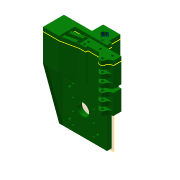
# Autodesk Inventor part: cellSTORM_cellphone_objectivelens_mount_flexure
Saved by Autodesk Inventor 2019 (Build 230136000, 136)
## iProperties
Created: 2020-02-11
Part Number: cellSTORM_cellphone_objectivelens_mount_flexure
Material: Generic
Document SubType Name: Modeling
Designer: diederichbenedict
Density: 1 g/cm^3
Appearance: Dark Green
Author: diederichbenedict
Autodesk Inventor part; units mm, degrees
ref_plane "YZ Plane" through (0, 0, 0) normal (1, 0, 0) x (0, 1, 0)
ref_plane "XZ Plane" through (0, 0, 0) normal (0, 1, 0) x (-1, 0, 0)
ref_plane "XY Plane" through (0, 0, 0) normal (0, 0, 1) x (1, 0, 0)
ref_plane "Work Plane1" through (0, 0, 0) normal (0, 0, 1) x (1, 0, 0)
sketch "Sketch1" plane through (0, 0, 0) normal (0, 0, 1) x (1, 0, 0)
  line L0 (28, 30) -> (30, 28) projected
  line L1 (28, 30) -> (-28, 30) projected
  line L2 (-30, 28) -> (-28, 30) projected
  line L3 (-30, 28) -> (-30, -28) projected
  line L4 (-28, -30) -> (-30, -28) projected
  line L5 (-28, -30) -> (28, -30) projected
  line L6 (30, -28) -> (28, -30) projected
  line L7 (30, -28) -> (30, 28) projected
  circle A0 centre (-17.5, -17.5) radius 1.95 projected
  circle A1 centre (17.5, 17.5) radius 1.95 projected
  circle A2 centre (17.5, -17.5) radius 1.95 projected
  circle A3 centre (-17.5, 17.5) radius 1.95 projected
  circle A4 centre (0, 0) radius 7.5 projected
  line L8 (-30, -30) -> (30, -30)
  line L9 (30, -30) -> (30, 30)
  line L10 (30, 30) -> (-30, 30)
  line L11 (-30, 30) -> (-30, -30)
  line L12 (30, 30) -> (-30, 30)
  line L13 (-30, 30) -> (-30, 45)
  line L14 (-30, 45) -> (30, 45)
  line L15 (30, 45) -> (30, 30)
  circle A5 centre (-13, 22.5) radius 1.45
  circle A6 centre (-13, 7.5) radius 1.45
  circle A7 centre (-13, -7.5) radius 1.45
  circle A8 centre (-13, -22.5) radius 1.45
  circle A9 centre (13, -22.5) radius 1.45
  circle A10 centre (13, 22.5) radius 1.45
  circle A11 centre (13, 7.5) radius 1.45
  circle A12 centre (13, -7.5) radius 1.45
  point P0 (0, 0)
  dimension "d2" = 60
  dimension "d3" = 15
  constraints: 16 end point, 8 centre point, 4 parallel, 2 horizontal, 2 perpendicular, 16 other
  measures "d2" distance of L13.end L14.end
  measures "d3" distance of L12.end L13.end
extrude "Extrusion1" add sketch "Sketch1" along normal blind 6
sketch "Sketch2" plane through (-30, 45, 0) normal (0, 1, 0) x (1, 0, 0)
  line L0 (60, 0) -> (0, 0) projected
  line L1 (0, 0) -> (0, -6) projected
  line L2 (60, -6) -> (0, -6) projected
  line L3 (60, 0) -> (60, -6) projected
  line L4 (0, 0) -> (0, -6) projected
  line L5 (0, 0) -> (19.8609, 0)
  line L6 (19.8609, 0) -> (19.8609, -26.2545)
  line L7 (19.8609, 0) -> (60, 0)
  line L8 (60, 0) -> (60, -6)
  line L9 (60, -6) -> (19.8609, -6)
  line L10 (19.8609, -6) -> (19.8609, 0)
  line L11 (19.8599, -13.0545) -> (19.8609, -13.4545)
  line L12 (41, -13.4) -> (41, -13)
  line L13 (41, -21.8) -> (49, -21.8)
  line L14 (49, -21.8) -> (49, -9)
  line L15 (49, -9) -> (41, -9)
  line L16 (41, -9.511) -> (41, -21.289)
  line L17 (49, -9) -> (81, -9) construction
  line L18 (81, -9) -> (81, -19) construction
  line L19 (81, -19) -> (49, -19) construction
  line L20 (49, -19) -> (49, -9) construction
  line L21 (49, -9) -> (81, -9)
  line L22 (81, -9) -> (81, -19)
  line L23 (81, -19) -> (49, -19)
  line L24 (49, -19) -> (49, -9)
  line L25 (41, -21.8) -> (41, -21.4)
  line L26 (19.8609, -25.4) -> (19.8609, -26.2545)
  circle A0 centre (45, -19) radius 1.4
  circle A1 centre (45, -14) radius 1.4
  circle A2 centre (75, -14) radius 1.4
  circle A3 centre (60, -14) radius 1.4
  line L27 (0, 0) -> (0, -6) projected
  line L28 (0, -6) -> (19.8609, -6)
  line L29 (19.8609, -6) -> (19.8609, -26.2545)
  line L30 (19.8609, -26.2545) -> (0, -26.2545)
  line L31 (0, -26.2545) -> (0, -6)
  line L32 (41, -21.8) -> (19.8609, -26.2545)
  line L33 (41, -9) -> (19.8609, -13.4545)
  line L34 (22.8609, -25.1114) -> (22.1392, -21.6866)
  line L35 (22.1392, -21.6866) -> (36.8169, -18.5936)
  line L36 (36.8169, -18.5936) -> (37.5386, -22.0184)
  line L37 (24.8765, -24.6866) -> (22.8609, -25.1114)
  line L38 (22.5001, -13.4094) -> (23.2218, -16.8342)
  line L39 (23.2218, -16.8342) -> (37.8994, -13.7412)
  line L40 (37.8994, -13.7412) -> (37.1778, -10.3164)
  line L41 (19.8609, -13.9655) -> (22.5001, -13.4094)
  line L42 (37.1778, -10.3164) -> (41, -9.511)
  line L43 (19.8609, -25.7436) -> (22.8609, -25.1114)
  line L44 (37.5386, -22.0184) -> (41, -21.289)
  point P0 (30, 0)
  dimension "d22" = 0.4
  dimension "d27" = 8
  dimension "d32" = 32
  dimension "d33" = 10
  dimension "d35" = 0.4
  dimension "d46" = 49
  dimension "d48" = 2.8
  dimension "d50" = 2.8
  dimension "d51" = 2.8
  dimension "d52" = 2.8
  dimension "d53" = 6
  dimension "d54" = 5
  dimension "d55" = 15
  dimension "d56" = 15
  dimension "d57" = 0
  dimension "d58" = 0
  dimension "d59" = 5
  dimension "d95" = 12.8
  dimension "d96" = 3
  dimension "d99" = 3.5
  dimension "d100" = 15
  dimension "d101" = 3
  dimension "d102" = 3.5
  dimension "d103" = 15
  dimension "d104" = 0.5
  constraints: 78 end point, 22 parallel, 12 perpendicular, 6 horizontal, 5 point on line, 4 centre point
  measures "d22" distance of L12.end L12.start
  measures "d27" distance between parallel lines of L14 L16
  measures "d32" distance of L18.end L19.end
  measures "d33" distance of L17.end L18.end
  measures "d35" distance of L25.end L13.start
  measures "d46" distance between parallel lines of L1 L20
  measures "d48" diameter of A0
  measures "d50" diameter of A1
  measures "d51" diameter of A2
  measures "d52" diameter of A3
  measures "d53" distance from line of A2.centre L18
  measures "d54" distance from line of A2.centre L17
  measures "d55" distance of A2.centre A3.centre
  measures "d56" distance of A1.centre A3.centre
  measures "d57" horizontal distance of A1.centre A0.centre
  measures "d58" vertical distance of A2.centre A3.centre
  measures "d59" distance of A1.centre A0.centre
  measures "d95" distance between parallel lines of L13 L15
  measures "d96" distance between parallel lines of L15 L9
  measures "d99" distance between parallel lines of L37 L35
  measures "d100" distance between parallel lines of L36 L34
  measures "d101" horizontal distance of L43.start L34.start
  measures "d102" distance of L38.start L38.end
  measures "d103" distance of L39.end L38.end
  measures "d104" distance between parallel lines of L42 L33
extrude "Extrusion2" add sketch "Sketch2" along normal blind 35 contours L3 L2 L6 L0 | L6 L2 L1 L0 | L6 L30 L31 L2 | L33 L15 L14 L13 L32 L6 L43 L34 L35 L36 L44 L16 L12 L42 L40 L39 L38 L41 | L21 L22 L23 L14
sketch "Sketch3" plane through (-30, -30, 0) normal (-1, 0, 0) x (0, 0, 1)
  line L0 (0, 0) -> (0, 110) projected
  line L1 (0, 0) -> (6, 0) projected
  line L2 (6, 75) -> (6, 0) projected
  line L3 (26.2545, 75) -> (6, 0)
  line L4 (6, 75) -> (26.2545, 75) projected
  line L5 (26.2545, 75) -> (26.2545, 110) projected
  line L6 (0, 110) -> (26.2545, 110) projected
  line L7 (6, 0) -> (6, 75)
  line L8 (6, 0) -> (6, 110) projected
  line L9 (6, 75) -> (26.2545, 75)
  point P0 (0, 30)
  constraints: 6 end point, 2 collinear
extrude "Extrusion3" add sketch "Sketch3" against normal blind 5
sketch "Sketch4" plane through (0, 0, 0) normal (0, 0, -1) x (-1, 0, 0)
  circle A0 centre (-15.9426, 57.924) radius 3.2 construction
  circle A1 centre (-15.9426, 60.1479) radius 4.5 construction
  circle A2 centre (-15.9426, 60.1479) radius 3.2
  circle A3 centre (-15.9426, 60.1479) radius 4.3038
  point P0 (0, 0)
  dimension "d90" = 6.4
  constraints: 3 centre point, 1 coincident
  measures "d90" diameter of A2
extrude "Extrusion4" cut sketch "Sketch4" against normal up to surface (6 mm away) contours A2 | A3
sketch "Sketch5" plane through (0, 0, 0) normal (0, 0, -1) x (-1, 0, 0)
  circle A0 centre (-15.9426, 57.924) radius 7.26 construction
  circle A1 centre (-15.9426, 57.924) radius 4.5878 construction
  circle A2 centre (-15.9426, 57.924) radius 7.26 construction
  circle A3 centre (-15.9426, 57.924) radius 6.335 construction
  line L0 (-26.6781, 61.3895) -> (-26.6781, 80)
  line L1 (-51, 80) -> (7, 80) projected
  line L2 (-5.1355, 60.1479) -> (-5.1355, 80)
  line L3 (-8, 80) -> (7, 80) projected
  circle A4 centre (-15.9426, 60.1479) radius 6.45
  circle A5 centre (-15.9426, 60.1479) radius 10.8071
  point P0 (0, 0)
  dimension "d88" = 12.9
  dimension "d89" = 0
  constraints: 4 end point, 2 centre point, 2 point on circle, 2 point on line, 2 vertical, 1 coincident, 1 tangent
  measures "d88" diameter of A4
  measures "d89" horizontal distance of A0.centre A4.centre
extrude "Extrusion5" add sketch "Sketch5" along normal blind 14
sketch "Sketch6" plane through (-30, 45, 0) normal (0, -1, 0) x (1, 0, 0)
  line L0 (19.8609, 6) -> (5, 6) projected
  line L1 (81, 19) -> (81, 9) projected
  line L2 (49, 19) -> (81, 19) projected
  line L3 (49, 21.8) -> (49, 19) projected
  line L4 (49, 21.8) -> (49, 19) projected
  line L5 (81, 9) -> (49, 9)
  line L6 (49, 9) -> (49, 19)
  line L7 (49, 19) -> (81, 19)
  line L8 (81, 19) -> (81, 9)
  line L9 (19.8609, 13.4545) -> (19.8609, 6) projected
  line L10 (41, 21.8) -> (49, 21.8) projected
  line L11 (81, 9) -> (41, 9) projected
  line L12 (19.8609, 26.2545) -> (41, 21.8) projected
  line L13 (5, 26.2545) -> (19.8609, 26.2545) projected
  line L14 (41, 9) -> (19.8609, 13.4545) projected
  line L15 (5, 26.2545) -> (5, 6) projected
  point P0 (30, 0)
  constraints: 8 end point, 2 parallel, 1 horizontal, 1 perpendicular
extrude "Extrusion6" add sketch "Sketch6" along normal blind 20 contours L6 L2 L1 L5
sketch "Sketch7" plane through (-30, 80, 0) normal (0, 1, 0) x (1, 0, 0)
  line L0 (49, -21.8) -> (49, -19) projected
  line L1 (49, -19) -> (81, -19) projected
  line L2 (81, -19) -> (81, -9) projected
  line L3 (0, 0) -> (0, -26.2545) projected
  arc A0 (68.6392, -25.4245) -> (75.056, -24.1906) centre (71.5, -23) ccw
  line L4 (63.1946, -19) -> (68.6392, -25.4245)
  line L5 (49, -19) -> (81, -19) projected
  line L6 (81, -19) -> (63.1946, -19)
  line L7 (35.1355, 0) -> (0, 0) projected
  line L8 (19.8609, -13.4545) -> (19.8609, -6) projected
  line L9 (19.8609, -6) -> (60, -6) projected
  line L10 (60, -6) -> (60, 0) projected
  line L11 (41, -21.8) -> (49, -21.8) projected
  line L12 (60, 0) -> (56.6781, 0) projected
  line L13 (56.6781, 0) -> (56.6781, 14) projected
  line L14 (35.1355, 14) -> (56.6781, 14) projected
  line L15 (35.1355, 0) -> (35.1355, 14) projected
  line L16 (81, -9) -> (41, -9) projected
  line L17 (19.8609, -26.2545) -> (41, -21.8) projected
  line L18 (41, -9) -> (19.8609, -13.4545) projected
  line L19 (0, -26.2545) -> (19.8609, -26.2545) projected
  circle A1 centre (71.5, -23) radius 1.5
  line L20 (75.056, -24.1906) -> (75.8344, -20.6777) construction
  line L21 (75.8344, -20.6777) -> (78.0391, -19.411) construction
  line L22 (78.0391, -19.411) -> (81, -19) construction
  spline S0 degree 3 poles (75.056, -24.1906) (75.8344, -20.6777) (78.0391, -19.411) (81, -19) knots 1 1 1 1 2 2 2 2
  line L23 (63.1946, -19) -> (81, -19)
  point P0 (30, 0)
  point P1 (75.1208, -23.9758)
  dimension "d113" = 3
  dimension "d114" = 3.75
  dimension "d116" = 9.5
  dimension "d117" = 4
  constraints: 6 end point, 3 point on circle, 3 point on line, 2 centre point, 2 coincident, 2 horizontal, 1 collinear, 1 tangent, 5 other
  measures "d113" diameter of A1
  measures "d114" radius of A0
  measures "d116" distance from line of A0.centre L2
  measures "d117" distance from line of A0.centre L1
extrude "Extrusion7" add sketch "Sketch7" against normal blind 5 contours L1 S0 A0 L4
pattern_linear "Rectangular Pattern1" count 6 spacing 10 along (0, -1, 0) of "Extrusion7"
sketch "Sketch8" plane through (-30, 80, 0) normal (0, 1, 0) x (1, 0, 0)
  circle A0 centre (45, -19) radius 1.4 projected
  circle A1 centre (45, -14) radius 1.4 projected
  circle A2 centre (60, -14) radius 1.4 projected
  circle A3 centre (75, -14) radius 1.4 projected
  line L0 (49, -21.8) -> (49, -19) projected
  line L1 (49, -19) -> (63.1946, -19) projected
  line L2 (81, -19) -> (81, -9) projected
  line L3 (35.1355, 0) -> (0, 0) projected
  line L4 (0, 0) -> (0, -26.2545) projected
  circle A4 centre (45.9028, 5) radius 1.4
  line L5 (19.8609, -13.4545) -> (19.8609, -6) projected
  line L6 (19.8609, -6) -> (60, -6) projected
  line L7 (60, -6) -> (60, 0) projected
  line L8 (41, -21.8) -> (49, -21.8) projected
  line L9 (60, 0) -> (56.6781, 0) projected
  line L10 (56.6781, 0) -> (56.6781, 14) projected
  line L11 (35.1355, 14) -> (56.6781, 14) projected
  line L12 (35.1355, 0) -> (35.1355, 14) projected
  line L13 (81, -9) -> (41, -9) projected
  line L14 (19.8609, -26.2545) -> (41, -21.8) projected
  line L15 (41, -9) -> (19.8609, -13.4545) projected
  line L16 (0, -26.2545) -> (19.8609, -26.2545) projected
  line L17 (63.1946, -19) -> (68.6392, -25.4245) projected
  arc A5 (68.6392, -25.4245) -> (75.056, -24.1906) centre (71.5, -23) ccw projected
  point P0 (30, 0)
  dimension "d60" = 2.8
  constraints: 1 centre point, 1 other
  measures "d60" diameter of A4
sketch "Sketch9" plane through (-10.1391, 45, 12.9) normal (1, 0, 0) x (0, 0, -1)
  line L0 (-13.3545, 0) -> (6.9, 0) projected
  line L1 (12.9, -75) -> (12.9, 35) projected
  line L2 (12.9, -75) -> (6.9, -75) projected
  line L3 (6.9, -75) -> (-13.3545, 0) projected
  line L4 (-13.3545, 0) -> (-13.3545, 35) projected
  line L5 (12.9, 35) -> (-13.3545, 35) projected
  line L6 (6.9, 0) -> (6.9, -75) projected
  line L7 (6.9, -23.95) -> (6.9, -21.05) projected
  line L8 (12.9, -21.05) -> (12.9, -23.95) projected
  line L9 (6.9, -23.95) -> (6.9, -21.05) projected
  line L10 (-13.3545, 0) -> (6.9, -20.4113)
  line L11 (6.9, 0) -> (6.9, -20.4113)
  line L12 (12.9, -75) -> (12.9, 35) projected
  line L13 (-13.3545, 0) -> (6.9, 0)
  point P0 (12.9, -45)
  constraints: 6 end point, 1 parallel, 1 perpendicular, 1 point on line
extrude "Extrusion9" add sketch "Sketch9" against normal blind 4.5 contours L0 L6 L10
ref_plane "Work Plane2" through (11, 85, -38.3865) normal (0, -1, 0) x (1, 0, 0)
sketch "Sketch10" plane through (-30, 80, 0) normal (0, 1, 0) x (1, 0, 0)
  arc A0 (54.8484, -57.7591) -> (49, -21.8) centre (41.6525, -41.4501) ccw
  line L0 (75.6971, -30.7014) -> (75.6971, -57.7591)
  line L1 (75.6971, -57.7591) -> (54.8484, -57.7591)
  line L2 (19.8609, -13.9655) -> (22.5001, -13.4094) projected
  line L3 (22.5001, -13.4094) -> (23.2218, -16.8342) projected
  line L4 (23.2218, -16.8342) -> (37.8994, -13.7412) projected
  line L5 (37.8994, -13.7412) -> (37.1778, -10.3164) projected
  line L6 (37.1778, -10.3164) -> (41, -9.511) projected
  line L7 (41, -9.511) -> (41, -21.289) projected
  line L8 (41, -21.289) -> (37.5386, -22.0184) projected
  line L9 (37.5386, -22.0184) -> (36.8169, -18.5936) projected
  line L10 (36.8169, -18.5936) -> (22.1392, -21.6866) projected
  line L11 (22.1392, -21.6866) -> (22.8609, -25.1114) projected
  line L12 (22.8609, -25.1114) -> (19.8609, -25.7436) projected
  line L13 (19.8609, -13.9655) -> (19.8609, -25.7436) projected
  circle A1 centre (45, -14) radius 1.4 projected
  circle A2 centre (45, -19) radius 1.4 projected
  line L14 (0, -26.2545) -> (19.8609, -26.2545) projected
  line L15 (19.8609, -26.2545) -> (41, -21.8) projected
  line L16 (41, -21.8) -> (49, -21.8) projected
  line L17 (49, -21.8) -> (49, -19) projected
  line L18 (49, -19) -> (63.1946, -19) projected
  line L19 (81, -19) -> (81, -9) projected
  line L20 (81, -9) -> (41, -9) projected
  line L21 (41, -9) -> (19.8609, -13.4545) projected
  line L22 (19.8609, -13.4545) -> (19.8609, -6) projected
  line L23 (19.8609, -6) -> (60, -6) projected
  line L24 (60, -6) -> (60, 0) projected
  line L25 (60, 0) -> (56.6781, 0) projected
  line L26 (56.6781, 0) -> (56.6781, 14) projected
  line L27 (35.1355, 14) -> (56.6781, 14) projected
  line L28 (35.1355, 0) -> (35.1355, 14) projected
  line L29 (35.1355, 0) -> (0, 0) projected
  line L30 (0, 0) -> (0, -26.2545) projected
  circle A3 centre (60, -14) radius 1.4 projected
  circle A4 centre (75, -14) radius 1.4 projected
  line L31 (19.8609, -13.9655) -> (22.5001, -13.4094) projected
  line L32 (22.5001, -13.4094) -> (23.2218, -16.8342) projected
  line L33 (23.2218, -16.8342) -> (37.8994, -13.7412) projected
  line L34 (37.8994, -13.7412) -> (37.1778, -10.3164) projected
  line L35 (37.1778, -10.3164) -> (41, -9.511) projected
  line L36 (41, -9.511) -> (41, -21.289) projected
  line L37 (41, -21.289) -> (37.5386, -22.0184) projected
  line L38 (37.5386, -22.0184) -> (36.8169, -18.5936) projected
  line L39 (36.8169, -18.5936) -> (22.1392, -21.6866) projected
  line L40 (22.1392, -21.6866) -> (22.8609, -25.1114) projected
  line L41 (22.8609, -25.1114) -> (19.8609, -25.7436) projected
  line L42 (19.8609, -13.9655) -> (19.8609, -25.7436) projected
  circle A5 centre (45, -14) radius 1.4 projected
  circle A6 centre (45, -19) radius 1.4 projected
  line L43 (0, -26.2545) -> (19.8609, -26.2545) projected
  line L44 (19.8609, -26.2545) -> (41, -21.8) projected
  line L45 (41, -21.8) -> (49, -21.8) projected
  line L46 (49, -21.8) -> (49, -19) projected
  line L47 (49, -19) -> (63.1946, -19) projected
  line L48 (81, -19) -> (81, -9) projected
  line L49 (81, -9) -> (41, -9) projected
  line L50 (41, -9) -> (19.8609, -13.4545) projected
  line L51 (19.8609, -13.4545) -> (19.8609, -6) projected
  line L52 (19.8609, -6) -> (60, -6) projected
  line L53 (60, -6) -> (60, 0) projected
  line L54 (60, 0) -> (56.6781, 0) projected
  line L55 (56.6781, 0) -> (56.6781, 14) projected
  line L56 (35.1355, 14) -> (56.6781, 14) projected
  line L57 (35.1355, 0) -> (35.1355, 14) projected
  line L58 (35.1355, 0) -> (0, 0) projected
  line L59 (0, 0) -> (0, -26.2545) projected
  circle A7 centre (60, -14) radius 1.4 projected
  circle A8 centre (75, -14) radius 1.4 projected
  line L60 (19.8609, -13.4545) -> (19.8609, -13.9655)
  line L61 (19.8609, -25.7436) -> (22.8609, -25.1114) projected
  line L62 (19.8609, -25.7436) -> (19.8609, -26.2545)
  line L63 (63.1946, -19) -> (68.6392, -25.4245) projected
  arc A9 (68.6392, -25.4245) -> (75.056, -24.1906) centre (71.5, -23) ccw projected
  spline S0 degree 3 poles (75.056, -24.1906) (75.8344, -20.6777) (78.0391, -19.411) (81, -19) knots 0 0 0 0 1 1 1 1 projected
  line L64 (63.1946, -19) -> (68.6392, -25.4245) projected
  arc A10 (68.6392, -25.4245) -> (75.056, -24.1906) centre (71.5, -23) ccw projected
  arc A11 (33.1525, -71.4501) -> (36.6525, -74.9501) centre (36.6525, -71.4501) ccw projected
  line L65 (95.5325, -74.9501) -> (36.6525, -74.9501) projected
  arc A12 (95.5325, -74.9501) -> (99.0325, -71.4501) centre (95.5325, -71.4501) ccw projected
  line L66 (99.0325, 68.5499) -> (99.0325, -71.4501) projected
  arc A13 (99.0325, 68.5499) -> (95.5325, 72.0499) centre (95.5325, 68.5499) ccw projected
  line L67 (36.6525, 72.0499) -> (95.5325, 72.0499) projected
  arc A14 (36.6525, 72.0499) -> (33.1525, 68.5499) centre (36.6525, 68.5499) ccw projected
  line L68 (33.1525, -71.4501) -> (33.1525, 68.5499) projected
  circle A15 centre (71.5, -23) radius 1.5 projected
  constraints: 8 end point, 2 point on circle, 2 vertical, 1 centre point, 1 perpendicular, 2 other
extrude "Extrusion10" add sketch "Sketch10" along normal up to surface (5 mm away) contours L60 L21 L68 L4 L3 L2 | L13 L62 L14 L30 L29 L68 L23 L22 L60 | L12 L11 L10 L68 L15 L62 | L21 L20 L19 S0 A9 L63 L18 L17 L16 L15 L68 L10 L9 L8 L7 L6 L5 L4 | L68 L29 L28 L27 L26 L25 L24 L23
sketch "Sketch11" plane through (-30, 80, 0) normal (0, 1, 0) x (1, 0, 0)
  line L0 (41, -21.8) -> (49, -21.8)
  line L1 (52.2776, 11.65) -> (39.6076, 11.65)
  spline S0 degree 3 poles (35, -46.9) (34.8191, -46.9) (34.6301, -46.863) (34.287, -46.7191) (34.1324, -46.6123) (33.8883, -46.3682) (33.781, -46.2134) (33.6368, -45.8695) (33.6, -45.6801) (33.6, -45.3199) (33.6368, -45.1305) (33.781, -44.7866) (33.8883, -44.6318) (34.1324, -44.3877) (34.287, -44.2809) (34.6301, -44.137) (34.8191, -44.1) (35, -44.1) knots 0 0 0 0 0.12529 0.12529 0.250579 0.250579 0.37529 0.37529 0.5 0.5 0.62471 0.62471 0.749421 0.749421 0.87471 0.87471 1 1 1 1
  line L2 (45.55, 0) -> (49.45, 0)
  line L3 (14.45, 0) -> (10.55, 0)
  circle A0 centre (38, -3) radius 1.7
  circle A1 centre (56.6701, -3) radius 1.7
  circle A2 centre (3.0233, -3) radius 1.7
  line L4 (41, -9.511) -> (41, -21.289)
  line L5 (49, -19) -> (63.1946, -19)
  line L6 (63.1946, -19) -> (74.8156, -28.9469)
  arc A3 (74.8156, -28.9469) -> (81, -25.922) centre (77.2541, -26.098) ccw
  line L7 (81, -25.922) -> (81, -9)
  line L8 (81, -9) -> (41, -9)
  line L9 (19.8609, -26.2545) -> (41, -21.8)
  line L10 (49, -21.8) -> (49, -19)
  line L11 (41, -9) -> (19.8609, -13.4545)
  line L12 (19.8609, -13.9655) -> (22.5001, -13.4094)
  line L13 (22.5001, -13.4094) -> (23.2218, -16.8342)
  line L14 (23.2218, -16.8342) -> (37.8994, -13.7412)
  line L15 (37.8994, -13.7412) -> (37.1778, -10.3164)
  line L16 (37.1778, -10.3164) -> (41, -9.511)
  line L17 (41, -21.289) -> (37.5386, -22.0184)
  line L18 (37.5386, -22.0184) -> (36.8169, -18.5936)
  line L19 (36.8169, -18.5936) -> (22.1392, -21.6866)
  line L20 (22.1392, -21.6866) -> (22.8609, -25.1114)
  line L21 (22.8609, -25.1114) -> (19.8609, -25.7436)
  line L22 (19.8609, -25.7436) -> (19.8609, -26.2545)
  line L23 (19.8609, -13.4545) -> (19.8609, -13.9655)
  point P0 (30, 0)
  dimension "d75" = 3.4
  dimension "d76" = 3.4
  dimension "d77" = 3.4
  constraints: 3 centre point
  measures "d75" diameter of A0
  measures "d76" diameter of A1
  measures "d77" diameter of A2
extrude "Extrusion11" cut sketch "Sketch11" against normal through all contours A1 | A2
sketch "Sketch12" plane through (45.056, 50, 24.1906) normal (0, 1, 0) x (-0.7628894, 0, 0.6465291)
  arc A0 (0.2541, -0.176) -> (-7.7459, -0.176) centre (-3.7459, -0.176) ccw projected
  line L0 (-39.7434, -0.6261) -> (-7.7459, -0.6261) projected
  line L1 (-7.7459, -0.6261) -> (-7.7459, -0.176) projected
  arc A1 (5.693, -16.3009) -> (-14.0564, -16.7963) centre (-4.1817, -16.5486) ccw
  line L2 (-14.0564, -16.7963) -> (-17.116, -0.4229)
  line L3 (-17.116, -0.4229) -> (7.7636, 1.4774)
  line L4 (7.7636, 1.4774) -> (7.6982, -9.7156)
  line L5 (7.6982, -9.7156) -> (5.693, -16.3009)
  line L6 (5.693, -3.2074) -> (5.693, -11.6286) projected
  point P0 (18.7328, -47.5848)
  constraints: 8 end point, 2 point on circle, 1 centre point, 1 point on line
ref_plane "Work Plane3" through (38.05, 54.5, 23.5) normal (0, 1, 0) x (0, 0, 1)
extrude "Extrusion12" cut sketch "Sketch12" along normal up to surface (4.5 mm away) contours L3 L4 L5 A1 L2 L0 L1 A0 | A0 L1 L0 L2 L3
sketch "Sketch13" plane through (-10.1391, 85, 6) normal (0, 1, 0) x (1, 0, 0)
  line L0 (19.6316, 6) -> (19.6316, 20) projected
  line L1 (32.5316, 6) -> (32.5316, 20) projected
  circle A0 centre (26.0234, 10.5433) radius 1.49
  point P0 (10.1391, 6)
  dimension "d105" = 2.98
  constraints: 1 centre point
  measures "d105" diameter of A0
hole "Hole2" at (15.8843, 85, -4.5433) direction (0, -1, 0) diameter 2.8 end through all counterbore diameter 7 counterbore depth 7
sketch "Sketch14" plane through (0, 0, -14) normal (0, 0, -1) x (-1, 0, 0)
  arc A0 (-26.6781, 61.3895) -> (-5.1355, 60.1479) centre (-15.9426, 60.1479) ccw projected
  line L0 (-7.8994, 45) -> (-7.8994, 85) projected
  line L1 (-7.8994, 52.9298) -> (-23.9857, 52.9298)
  point P0 (0, 0)
  constraints: 2 end point, 2 point on circle, 1 horizontal, 1 point on line
extrude "Extrusion13" cut sketch "Sketch14" against normal up to surface (14 mm away)
sketch "Sketch15" plane through (0, 0, -14) normal (0, 0, -1) x (-1, 0, 0)
  line L0 (-19, 45) -> (-19, 85) projected
  line L1 (-11, 45) -> (-11, 85) projected
  line L2 (-9.9426, 75.1974) -> (-21.9426, 75.1974)
  line L3 (-21.9426, 75.1974) -> (-21.9426, 68.1974)
  line L4 (-21.9426, 68.1974) -> (-9.9426, 68.1974)
  line L5 (-9.9426, 68.1974) -> (-9.9426, 75.1974)
  line L6 (-9.9426, 75.1974) -> (-21.9426, 68.1974) construction
  line L7 (-21.9426, 75.1974) -> (-9.9426, 68.1974) construction
  circle A0 centre (-15.9426, 60.1479) radius 3.2 projected
  point P0 (0, 0)
  point P1 (-15.9426, 71.6974)
  dimension "d120" = 0
  dimension "d121" = 12
  dimension "d122" = 7
  constraints: 12 end point, 2 midpoint, 2 parallel, 1 horizontal, 1 perpendicular
  measures "d120" horizontal distance of A0.centre point (-15.943, 71.697)
  measures "d121" distance between parallel lines of L3 L5
  measures "d122" distance between parallel lines of L2 L4
extrude "Extrusion14" cut sketch "Sketch15" against normal up to surface (14 mm away) contours L4 L3 L2 L0 | L0 L2 L1 L4 | L1 L2 L5 L4
body "Solid1"
